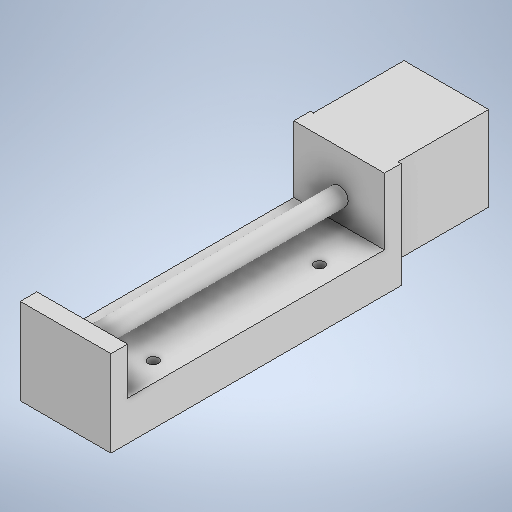
# Autodesk Inventor part: AE_50MM_STAGE
Saved by Autodesk Inventor 2025.2 (Build 292293000, 293)
## iProperties
Created: 2026-02-09
Part Number: AE_50MM_STAGE
Material: Generic
Document SubType Name: Modeling
Designer: composite
Density: 1 g/cm^3
Appearance: Default
Author: composite
Autodesk Inventor part; units mm, degrees
ref_plane "YZ Plane" through (0, 0, 0) normal (1, 0, 0) x (0, 1, 0)
ref_plane "XZ Plane" through (0, 0, 0) normal (0, 1, 0) x (-1, 0, 0)
ref_plane "XY Plane" through (0, 0, 0) normal (0, 0, 1) x (1, 0, 0)
sketch "Sketch1" plane through (0, 0, 0) normal (0, 1, 0) x (-1, 0, 0)
  line L0 (0, 0) -> (30, 0)
  line L1 (30, 0) -> (30, -96)
  line L2 (30, -96) -> (0, -96)
  line L3 (0, -96) -> (0, 0)
  dimension "d0" = 30
  dimension "d1" = 96
  constraints: 8 end point, 2 parallel, 1 horizontal, 1 perpendicular
  measures "d0" distance of L1.end L2.end
  measures "d1" distance of L0.end L1.end
extrude "Extrusion1" add sketch "Sketch1" along normal blind 13
sketch "Sketch2" plane through (0, 13, 0) normal (0, 1, 0) x (1, 0, 0)
  line L0 (-30, 96) -> (-30, 0) projected
  line L1 (0, 0) -> (0, 96) projected
  line L2 (-30, 0) -> (0, 0)
  line L3 (0, 0) -> (0, 5.5)
  line L4 (0, 5.5) -> (-30, 5.5)
  line L5 (-30, 5.5) -> (-30, 0)
  line L6 (0, 96) -> (-30, 96)
  line L7 (-30, 96) -> (-30, 90.5)
  line L8 (-30, 90.5) -> (0, 90.5)
  line L9 (0, 90.5) -> (0, 96)
  line L10 (-30, 96) -> (0, 96)
  line L11 (0, 96) -> (0, 90.5)
  line L12 (0, 90.5) -> (-30, 90.5)
  line L13 (-30, 90.5) -> (-30, 96)
  dimension "d4" = 5.5
  dimension "d5" = 5.5
  constraints: 24 end point, 6 parallel, 3 horizontal, 3 perpendicular, 2 point on line
  measures "d4" distance between parallel lines of L2 L4
  measures "d5" distance between parallel lines of L6 L8
extrude "Extrusion2" add sketch "Sketch2" along normal blind 15.5 contours L4 L1 L2 L0
sketch "Sketch4" plane through (0, 13, 0) normal (0, 1, 0) x (1, 0, 0)
  line L0 (0, 0) -> (0, 96) projected
  line L1 (-30, 96) -> (-30, 0) projected
  line L2 (0, 96) -> (-30, 96)
  line L3 (-30, 96) -> (-30, 90.5)
  line L4 (-30, 90.5) -> (0, 90.5)
  line L5 (0, 90.5) -> (0, 96)
  point P0 (0, 90.5)
  dimension "d8" = 5.5
  constraints: 8 end point, 2 parallel, 1 horizontal, 1 perpendicular, 1 point on line
  measures "d8" distance between parallel lines of L2 L4
extrude "Extrusion3" add sketch "Sketch4" along normal blind 22
sketch "Sketch6" plane through (0, 0, -96) normal (0, 0, -1) x (-1, 0, 0)
  line L0 (30, 35) -> (0, 35) construction
  line L1 (30, 0) -> (30, 28.5) projected
  line L2 (0, 35) -> (30, 35) construction
  line L3 (30, 35) -> (30, 7) construction
  line L4 (30, 7) -> (0, 7) construction
  line L5 (0, 7) -> (0, 35) construction
  line L6 (0, 7) -> (30, 35) construction
  line L7 (0, 35) -> (30, 7) construction
  circle A0 centre (15, 21) radius 3
  point P0 (0, 0)
  dimension "d11" = 28
  dimension "d12" = 6
  constraints: 12 end point, 2 parallel, 1 centre point, 1 horizontal, 1 midpoint, 1 perpendicular, 1 point on line
  measures "d11" distance between parallel lines of L0 L4
  measures "d12" diameter of A0
extrude "Extrusion4" add sketch "Sketch6" against normal up to surface (90.5 mm away)
sketch "Sketch7" plane through (0, 0, -96) normal (0, 0, -1) x (-1, 0, 0)
  line L0 (30, 0) -> (30, 28.5) projected
  line L1 (30, 35) -> (0, 35) projected
  line L2 (1, 35) -> (29, 35)
  line L3 (29, 35) -> (29, 7)
  line L4 (29, 7) -> (1, 7)
  line L5 (1, 7) -> (1, 35)
  point P0 (0, 0)
  point P1 (15, 35)
  dimension "d15" = 28
  constraints: 8 end point, 2 midpoint, 2 parallel, 2 perpendicular, 1 horizontal, 1 point on line
  measures "d15" distance of L4.end L2.start
extrude "Extrusion5" add sketch "Sketch7" along normal blind 30
sketch "Sketch8" plane through (0, 0, 0) normal (0, -1, 0) x (1, 0, 0)
  circle A0 centre (-6.5, -75.5) radius 1.7
  circle A1 centre (-23.5, -75.5) radius 1.7
  circle A2 centre (-6.5, -20.5) radius 1.7
  circle A3 centre (-23.5, -20.5) radius 1.7
  line L0 (0, 0) -> (0, -96) projected
  line L1 (-30, 0) -> (0, 0) projected
  line L2 (-30, -96) -> (-30, 0) projected
  line L3 (0, -96) -> (-30, -96) projected
  dimension "d18" = 3.4
  dimension "d19" = 55
  dimension "d20" = 6.5
  dimension "d21" = 20.5
  dimension "d22" = 6.5
  dimension "d25" = 17
  dimension "d26" = 20.5
  constraints: 4 centre point, 3 equal radius, 2 horizontal alignment, 2 vertical alignment
  measures "d18" diameter of A0
  measures "d19" distance of A3.centre A1.centre
  measures "d20" distance from line of A2.centre L0
  measures "d21" distance from line of L1 A2.centre
  measures "d22" distance from line of L2 A3.centre
  measures "d25" distance of A3.centre A2.centre
  measures "d26" distance from line of L3 A0.centre
extrude "Extrusion6" cut sketch "Sketch8" against normal blind 30 contours A0 | A1 | A2 | A3
equation "\"d5\" = d4"
equation "\"d22\" = d20"
body "Solid1"
